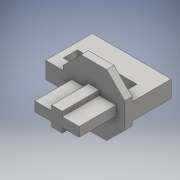
# Autodesk Inventor part: Replacement latch
Saved by Autodesk Inventor 2016 (Build 200138000, 138)
## iProperties
Created: 2016-08-29
Part Number: Replacement latch
Material: Generic
Document SubType Name: Modeling
Designer: andrew
Density: 1 g/cm^3
Appearance: Default
Author: andrew
Autodesk Inventor part; units mm, degrees
ref_plane "YZ Plane" through (0, 0, 0) normal (1, 0, 0) x (0, 1, 0)
ref_plane "XZ Plane" through (0, 0, 0) normal (0, 1, 0) x (-1, 0, 0)
ref_plane "XY Plane" through (0, 0, 0) normal (0, 0, 1) x (1, 0, 0)
sketch "Sketch1" plane through (0, 0, 0) normal (0, 0, 1) x (1, 0, 0)
  line L0 (-3.525, -2.075) -> (3.525, -2.075)
  line L1 (3.525, -2.075) -> (3.525, 2.075)
  line L2 (3.525, 2.075) -> (-3.525, 2.075)
  line L3 (-3.525, 2.075) -> (-3.525, -2.075)
  line L4 (-3.525, -2.075) -> (3.525, 2.075) construction
  line L5 (3.525, -2.075) -> (-3.525, 2.075) construction
  line L6 (-2.925, -1.1225) -> (2.405, -1.1225)
  line L7 (2.405, -1.1225) -> (2.405, 0.1475)
  line L8 (2.405, 0.1475) -> (-2.925, 0.1475)
  line L9 (-2.925, 0.1475) -> (-2.925, -1.1225)
  point P0 (0, 0)
  dimension "d0" = 4.15
  dimension "d1" = 7.05
  dimension "d2" = 5.33
  dimension "d3" = 0.6
  dimension "d4" = 1.27
  dimension "d5" = 0.9525
  constraints: 20 end point, 4 parallel, 2 horizontal, 2 midpoint, 2 perpendicular
  measures "d0" distance of L2.end L0.start
  measures "d1" distance of L1.end L2.end
  measures "d2" distance of L7.end L8.end
  measures "d3" distance between parallel lines of L3 L9
  measures "d4" distance of L6.end L7.end
  measures "d5" distance between parallel lines of L0 L6
extrude "Extrusion1" add sketch "Sketch1" along normal mid plane 1.5
sketch "Sketch2" plane through (-3.525, -2.075, 0.75) normal (0, -1, 0) x (1, 0, 0)
  line L0 (7.05, 0.3891) -> (7.05, -1.8891)
  line L1 (7.05, -1.8891) -> (5.4391, -3.5)
  line L2 (5.4391, -3.5) -> (3.1609, -3.5)
  line L3 (3.1609, -3.5) -> (1.55, -1.8891)
  line L4 (1.55, -1.8891) -> (1.55, 0.3891)
  line L5 (1.55, 0.3891) -> (3.1609, 2)
  line L6 (3.1609, 2) -> (5.4391, 2)
  line L7 (5.4391, 2) -> (7.05, 0.3891)
  line L8 (7.05, -1.5) -> (7.05, 0) projected
  line L9 (3.825, -0.33) -> (3.825, 0.1)
  line L10 (3.825, 0.1) -> (4.775, 0.1)
  line L11 (4.775, 0.1) -> (4.775, -0.33)
  line L12 (4.775, -0.33) -> (6.275, -0.33)
  line L13 (6.275, -0.33) -> (6.275, -1.17)
  line L14 (6.275, -1.17) -> (4.775, -1.17)
  line L15 (4.775, -1.17) -> (4.775, -1.6)
  line L16 (4.775, -1.6) -> (3.825, -1.6)
  line L17 (3.825, -1.6) -> (3.825, -1.17)
  line L18 (3.825, -1.17) -> (2.325, -1.17)
  line L19 (2.325, -1.17) -> (2.325, -0.33)
  line L20 (2.325, -0.33) -> (3.825, -0.33)
  line L21 (4.3, 0.1) -> (4.3, -1.6) construction
  line L22 (2.325, -0.75) -> (6.275, -0.75) construction
  point P0 (3.525, -0.75)
  point P1 (4.3, -0.75)
  dimension "d8" = 5.5
  dimension "d9" = 3.95
  dimension "d10" = 1.7
  dimension "d11" = 0.84
  dimension "d12" = 0.95
  constraints: 44 end point, 8 perpendicular, 6 midpoint, 6 point on line, 2 collinear, 1 horizontal alignment, 1 symmetric about line, 1 vertical, 19 other
  measures "d8" distance between parallel lines of L0 L4
  measures "d9" distance of L22.start L22.end
  measures "d10" distance of L21.start L21.end
  measures "d11" distance of L12.end L13.end
  measures "d12" distance of L9.end L10.end
extrude "Extrusion2" add sketch "Sketch2" against normal blind 0.65 contours L0 L1 L2 L3 L4 L5 L6 L7 | L9 L10 L11 L12 L13 L14 L15 L16 L17 L18 L19 L20
extrude "Extrusion3" add sketch "Sketch2" along normal blind 3.3 contours L9 L10 L11 L12 L13 L14 L15 L16 L17 L18 L19 L20
body "Solid1"
